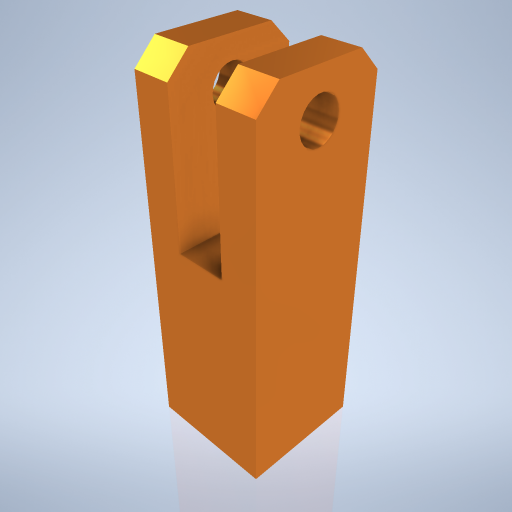
# Autodesk Inventor part: kopf
Saved by Autodesk Inventor 2024.2 (Build 282272000, 272)
## iProperties
Created: 2024-04-01
Part Number: kopf
Material: Generisch
Document SubType Name: Modeling
Designer: Fabri
Density: 1 g/cm^3
Appearance: Metall - 1600F (heiß)
Author: Fabri
Autodesk Inventor part; units mm, degrees
ref_plane "YZ Plane" through (0, 0, 0) normal (1, 0, 0) x (0, 1, 0)
ref_plane "XZ Plane" through (0, 0, 0) normal (0, 1, 0) x (-1, 0, 0)
ref_plane "XY Plane" through (0, 0, 0) normal (0, 0, 1) x (1, 0, 0)
sketch "Skizze1" plane through (0, 0, 0) normal (0, 0, 1) x (1, 0, 0)
  line L0 (-1.5, -1.5) -> (1.5, -1.5)
  line L1 (1.5, -1.5) -> (1.5, 1.5)
  line L2 (1.5, 1.5) -> (-1.5, 1.5)
  line L3 (-1.5, 1.5) -> (-1.5, -1.5)
  line L4 (-1.5, -1.5) -> (1.5, 1.5) construction
  line L5 (1.5, -1.5) -> (-1.5, 1.5) construction
  point P0 (0, 0)
  dimension "d0" = 3
  dimension "d1" = 3
  constraints: 12 end point, 2 midpoint, 2 parallel, 1 horizontal, 1 perpendicular
  measures "d0" distance of L2.end L1.end
  measures "d1" distance of L1.end L0.end
extrude "Extrusion1" add sketch "Skizze1" along normal blind 9
sketch "Skizze2" plane through (0, 0, 9) normal (0, 0, 1) x (1, 0, 0)
  line L0 (0, 0) -> (0, 3.7062) construction
  line L1 (1.5, 1.5) -> (-1.5, 1.5) projected
  line L2 (-0.6, -1.5) -> (0.6, -1.5)
  line L3 (0.6, -1.5) -> (0.6, 1.5)
  line L4 (0.6, 1.5) -> (-0.6, 1.5)
  line L5 (-0.6, 1.5) -> (-0.6, -1.5)
  line L6 (-1.5, -1.5) -> (1.5, -1.5) projected
  dimension "d4" = 1.2
  constraints: 10 end point, 2 parallel, 2 point on line, 1 horizontal, 1 perpendicular, 1 vertical, 1 other
  measures "d4" distance between parallel lines of L3 L5
extrude "Extrusion2" cut sketch "Skizze2" against normal blind 4
sketch "Skizze3" plane through (1.5, -1.5, 0) normal (1, 0, 0) x (0, 0, -1)
  line L0 (-9, 0) -> (-9, 3) projected
  line L1 (0, 0) -> (0, 3) projected
  point P0 (0, 1.5)
  point P1 (-8, 1.5)
  point P2 (-9, 1.5)
  dimension "d14" = 8
  constraints: 1 horizontal alignment, 1 midpoint
  measures "d14" distance from line of L1 point (-8, 1.5)
hole "Bohrung1" at (1.5, 0, 8) direction (-1, 0, 0) diameter 1 depth 0.9
mirror "Spiegeln1" about plane through (0, 0, 0) normal (1, 0, 0) of "Bohrung1"
sketch "Skizze4" plane through (0, 0, 0) normal (0, 0, -1) x (-1, 0, 0)
  line L0 (-1.5, -1.5) -> (-1.5, 1.5) projected
  line L1 (1.5, -1.5) -> (-1.5, -1.5) projected
  point P0 (0, 0)
  point P1 (0, 0)
  point P2 (-1.5, 0)
  point P3 (0, -1.5)
  constraints: 2 midpoint, 1 horizontal alignment, 1 vertical alignment
hole "Bohrung2" at (0, 0, 0) direction (0, 0, 1) diameter 1.5 depth 2.5 tip angle 118
chamfer "Fasen1" distance 0.5 angle 45 4 edges at (1.05, -1.5, 9) (1.05, 1.5, 9) (-1.05, 1.5, 9) (-1.05, -1.5, 9)
